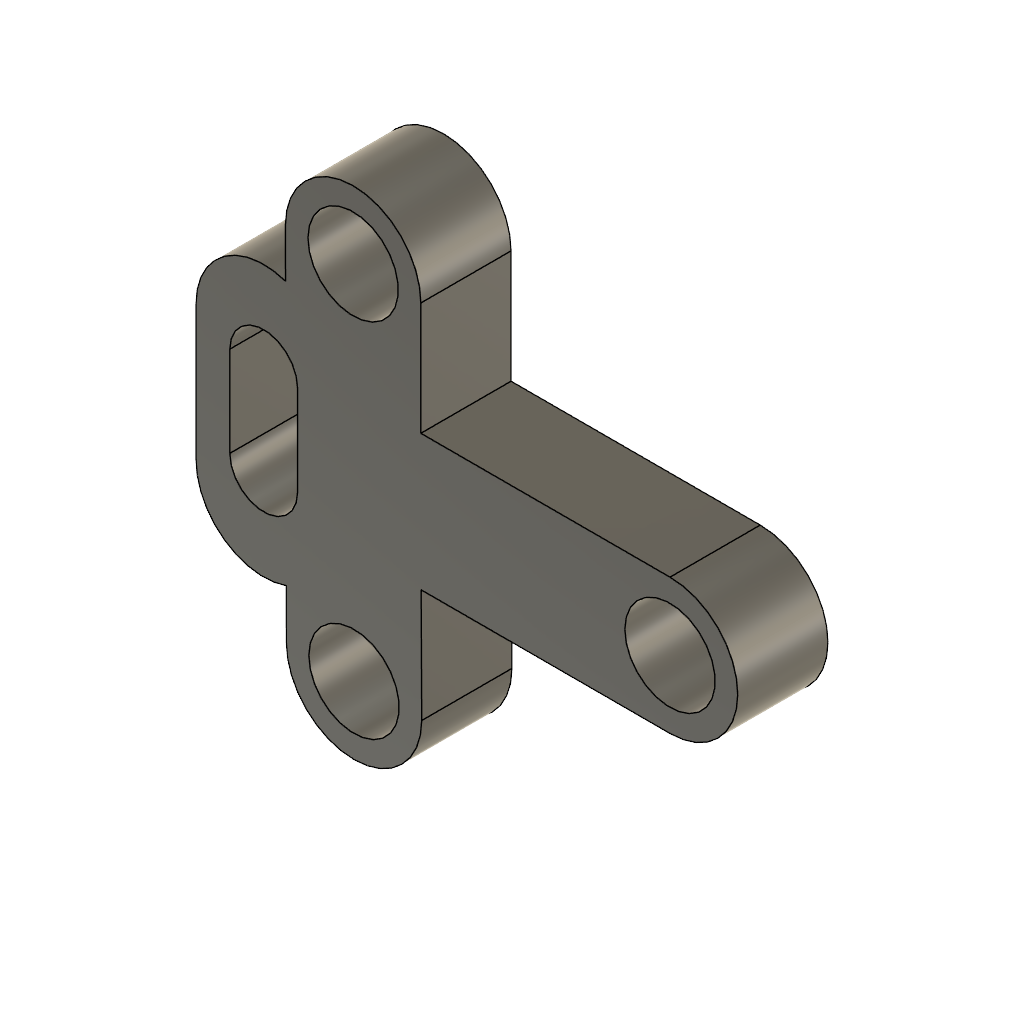
exercise 11 (Autodesk Fusion 360 design; units mm, degrees)
part number: 2026-10-06-22-45-53-690
Autodesk Fusion 360 part; units mm, degrees
sketch "Sketch1" plane through (0, 0, 0) normal (0, 1, 0) x (1, 0, 0)
  circle A0 centre (-0.1967, -80) radius 10
  circle A1 centre (-0.1967, -80) radius 5
  circle A2 centre (0, 0) radius 5
  circle A3 centre (0, 0) radius 10
  circle A4 centre (70, -40) radius 10
  circle A5 centre (70, -40) radius 5
  line L0 (-27.5, -30) -> (-27.5, -50)
  arc A6 (-27.5, -50) -> (-12.5, -50) centre (-20, -50) ccw
  line L1 (-12.5, -50) -> (-12.5, -30)
  arc A7 (-12.5, -30) -> (-27.5, -30) centre (-20, -30) ccw
  line L2 (-20, -30) -> (-20, -50) construction
  line L3 (-35, -25) -> (-35, -55)
  arc A8 (-35, -55) -> (-15.168, -69.2004) centre (-20, -55) ccw
  arc A9 (-15.0308, -10.847) -> (-35, -25) centre (-20, -25) ccw
  line L4 (-20, -25) -> (-20, -55) construction
  line L5 (70, -25) -> (14.8802, -25)
  line L6 (70, -55) -> (14.8033, -55)
  line L7 (-15, 0) -> (-15.0308, -10.847)
  line L8 (15, 0) -> (14.8802, -25)
  line L9 (14.8033, -80) -> (14.8033, -55)
  arc A10 (14.9993, -0.1437) -> (-15, 0) centre (0, 0) ccw
  line L10 (-15.1967, -79.96) -> (-15.168, -69.2004)
  arc A11 (-15.1967, -79.96) -> (14.8033, -80) centre (-0.1967, -80) ccw
  arc A12 (70, -55) -> (70, -25) centre (70, -40) ccw
  point P0 (-20, -40)
  point P1 (-20, -40)
  dimension "d1" = 30
  dimension "d2" = 20
  dimension "d3" = 10
  dimension "d4" = 10
  dimension "d5" = 20
  dimension "d6" = 30
  dimension "d7" = 30
  dimension "d8" = 20
  dimension "d9" = 10
  dimension "d10" = 15
  dimension "d11" = 20
  dimension "d12" = 80
  dimension "d13" = 70
  dimension "d14" = 40
  dimension "d15" = 20
  dimension "d16" = 30
  dimension "d17" = 30
  dimension "d18" = 30
  constraint concentric A0 A11
  constraint concentric A1 A11
  constraint coincident A2.centre A3.centre
  constraint concentric A3 A10
  constraint concentric A4 A12
  constraint concentric A5 A12
  constraint tangent L0 A6
  constraint tangent A6 L1
  constraint parallel L0 L1
  constraint tangent L1 A7
  constraint tangent L0 A7
  constraint vertical L2
  constraint midpoint L2 P1
  constraint tangent L3 A8
  constraint tangent L3 A9
  constraint parallel L2 L4
  constraint coincident P1 P0
  constraint midpoint L4 P1
  constraint vertical L9
  constraint tangent L10 A11
  constraint tangent L9 A11
  constraint tangent L5 A12
  constraint horizontal L5
  constraint tangent L6 A12
  constraint coincident L8.start A10
  constraint coincident L8 A10.start
  measures "d1" diameter of A11
  measures "d2" diameter of A0
  measures "d3" diameter of A1
  measures "d4" diameter of A2
  measures "d5" diameter of A3
  measures "d6" diameter of A10
  measures "d7" diameter of A12
  measures "d8" diameter of A4
  measures "d9" diameter of A5
  measures "d10" diameter of A6
  measures "d11" distance of A7.centre A6.centre
  measures "d12" vertical distance of A0.centre A2.centre
  measures "d13" horizontal distance of A2.centre A4.centre
  measures "d14" vertical distance of A0.centre A4.centre
  measures "d15" horizontal distance of A2.centre A7.centre
  measures "d16" vertical distance of A2.centre A7.centre
  measures "d17" diameter of A8
  measures "d18" distance of A9.centre A8.centre
extrude "Extrude1" add sketch "Sketch1" along normal blind 20 contours L3 A8 A9 L5 L6 L7 L8 L9 A10 L10 A11 A12
